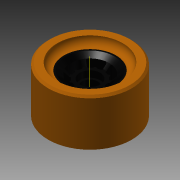
# Autodesk Inventor part: Wheel Blank Pro 83mm
Saved by Autodesk Inventor 2014 (Build 180170000, 170)
## iProperties
Created: 2014-05-15
Part Number: Wheel Blank Pro 83mm
Material: Polypropylene
Document SubType Name: Modeling
Designer: dliu
Density: 0.899 g/cm^3
Appearance: Orange
Author: dliu
Autodesk Inventor part; units mm, degrees
ref_plane "YZ Plane" through (0, 0, 0) normal (1, 0, 0) x (0, 1, 0)
ref_plane "XZ Plane" through (0, 0, 0) normal (0, 1, 0) x (-1, 0, 0)
ref_plane "XY Plane" through (0, 0, 0) normal (0, 0, 1) x (1, 0, 0)
sketch "Sketch2" plane through (0, 0, 0) normal (1, 0, 0) x (0, 1, 0)
  line L0 (0, 0) -> (0, 20.701) construction
  line L1 (0, 45) -> (26.035, 45)
  line L2 (26.035, 45) -> (26.035, 35.348)
  line L3 (18.415, 27.9864) -> (18.415, 26.204)
  line L4 (18.415, 26.204) -> (14.859, 20.701)
  line L5 (14.859, 20.701) -> (0, 20.701)
  arc A0 (26.035, 35.348) -> (18.415, 27.9864) centre (25.781, 27.9864) ccw
  line L6 (0, 20.701) -> (0, 45) construction
  line L7 (-36.449, 0) -> (36.449, 0) projected
  line L8 (0, 45) -> (-26.035, 45)
  line L9 (-26.035, 45) -> (-26.035, 35.348)
  line L10 (-18.415, 27.9864) -> (-18.415, 26.204)
  line L11 (-18.415, 26.204) -> (-14.859, 20.701)
  line L12 (-14.859, 20.701) -> (0, 20.701)
  arc A1 (-18.415, 27.9864) -> (-26.035, 35.348) centre (-25.781, 27.9864) ccw
  dimension "d0" = 45
  dimension "d2" = 9.652
  dimension "d4" = 11.176
  dimension "d6" = 20.701
  dimension "d7" = 7.366
  dimension "d9" = 26.035
  dimension "d10" = 7.3616
  dimension "d11" = 9.144
  constraints: 24 end point, 6 symmetric about line, 4 point on circle, 3 perpendicular, 2 centre point, 1 horizontal, 1 horizontal alignment, 1 vertical, 1 vertical alignment, 1 other
  measures "d0" distance of L0.start L1.start
  measures "d2" distance of L1.end L2.end
  measures "d4" distance from line of L2 L4.end
  measures "d6" distance from line of L0.start L5
  measures "d7" radius of A0
  measures "d9" distance between parallel lines of L2 L0
  measures "d10" vertical distance of L3.start L2.end
  measures "d11" vertical distance of L2.end L3.end
revolve "Revolution1" add sketch "Sketch2" angle 360 about axis through (0, -10, 0) along (0, 1, 0)
sketch "Sketch3" plane through (0, 0, 0) normal (0, 1, 0) x (-1, 0, 0)
  arc A0 (-1.905, 14.3521) -> (1.905, 14.3521) centre (0, 0) ccw
  circle A1 centre (0, 0) radius 10.9855
  circle A2 centre (0, 0) radius 8.4455
  circle A3 centre (0, 0) radius 20.701 projected
  line L0 (-1.905, 20.6132) -> (-1.905, 14.3521)
  line L1 (1.905, 20.6132) -> (1.905, 14.3521)
  arc A4 (1.905, 14.3521) -> (-1.905, 14.3521) centre (0, 0) ccw
  arc A5 (1.905, 20.6132) -> (-1.905, 20.6132) centre (0, 0) ccw
  dimension "d13" = 28.956
  dimension "d17" = 21.971
  dimension "d18" = 2.54
  dimension "d21" = 3.81
  constraints: 8 point on circle, 5 centre point, 4 end point, 3 coincident, 1 horizontal alignment, 1 parallel, 1 vertical
  measures "d13" diameter of A0
  measures "d17" diameter of A1
  measures "d18" radial gap between concentric circles of A2 A1
  measures "d21" distance between parallel lines of L1 L0
extrude "Bearing Holder" add sketch "Sketch3" along normal mid plane 21.1836 contours A4 A0
extrude "Bearing Holder Lip" add sketch "Sketch3" along normal mid plane 7.5184 contours A1
extrude "Spoke" add sketch "Sketch3" along normal up to surface (21.1836 mm away) from surface at -10.5918 contours L0 A3 L1 A4
chamfer "Chamfer1" distance 4.2672 distance2 4.572 2 edges at (0.9535, 10.5918, 20.679) (-0.9535, 10.5918, 20.679) measured on face at (0.9535, 11.0918, 20.679) measured on face at (-0.9535, 11.0918, 20.679)
chamfer "Chamfer2" distance 4.2672 distance2 4.572 2 edges at (0.9535, -10.5918, 20.679) (-0.9535, -10.5918, 20.679) measured on face at (0.9535, -11.0918, 20.679) measured on face at (-0.9535, -11.0918, 20.679)
fillet "Fillet1" radius 1.27 8 edges at (-1.905, 0, 14.3521) (1.905, 0, 14.3521) (1.905, -12.7253, 20.6132) (1.905, 0, 20.6132) (1.905, 12.7253, 20.6132) (-1.905, -12.7253, 20.6132) (-1.905, 0, 20.6132) (-1.905, 12.7253, 20.6132)
pattern_circular "Spoke Pattern" count 6 over 360 about axis through (0, -10, 0) along (0, 1, 0) of "Fillet1", "Spoke", "Chamfer1", "Chamfer2"
sketch "Sketch5" plane through (0, 0, 0) normal (0, 1, 0) x (-1, 0, 0)
  line L0 (0, 0) -> (0, 14.478) construction
  arc A0 (-1.905, 14.3521) -> (1.905, 14.3521) centre (0, 0) ccw construction
  arc A1 (1.905, 14.3521) -> (-1.905, 14.3521) centre (0, 0) ccw construction
  line L1 (0, 0) -> (10.3505, 17.9276) construction
  line L2 (6.2265, 13.0707) -> (6.9885, 14.3905)
  line L3 (6.9885, 14.3905) -> (8.9683, 13.2475)
  line L4 (8.9683, 13.2475) -> (8.2063, 11.9277)
  circle A2 centre (0, 0) radius 20.701 construction
  arc A3 (8.2063, 11.9277) -> (6.2265, 13.0707) centre (0, 0) ccw
  point P0 (7.9784, 13.819)
  dimension "d34" = 30
  dimension "d35" = 2.286
  dimension "d36" = 1.524
  constraints: 10 end point, 5 point on circle, 2 parallel, 1 centre point, 1 coincident, 1 midpoint, 1 perpendicular, 1 point on line, 1 vertical, 2 other
  measures "d34" angle of L1 L0
  measures "d35" distance of L2.end L3.end
  measures "d36" distance of L3.end L4.end
extrude "Nib" add sketch "Sketch5" against normal up to surface (21.1836 mm away) from surface at 10.5918
fillet "Fillet2" radius 1.27 2 edges at (-8.2063, 0, 11.9277) (-6.2265, 0, 13.0707)
fillet "Fillet3" radius 0.508 2 edges at (-6.9885, 0, 14.3905) (-8.9683, 0, 13.2475)
pattern_circular "Nib Pattern" count 6 over 360 about axis through (0, -10, 0) along (0, 1, 0) of "Nib", "Fillet2", "Fillet3"
chamfer "Wheel Inner Chamfer" distance 2.032 angle 45 1 edges at (0, 26.035, -45)
chamfer "Wheel Outer Chamfer" distance 2.032 distance2 7.4168 1 edges at (0, -26.035, -45) measured on face at (0, -25.535, -45)
body "Solid1"
